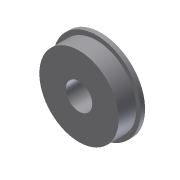
# Autodesk Inventor part: 375 ID 1125 OD flanged
Saved by Autodesk Inventor 2013 (Build 170138000, 138)
## iProperties
Created: 2011-07-15
Part Number: 375 ID 1125 OD flanged
Document SubType Name: Modeling
Designer: Dan Niemitalo
Density: 4.77592 g/cm^3
Mass: 31.751 g
Surface Area: 28.0121 cm^2
Volume: 6.64815 cm^3
Material: Generic
Author: Dan Niemitalo
Autodesk Inventor part; units mm, degrees
ref_plane "YZ Plane" through (0, 0, 0) normal (1, 0, 0) x (0, 1, 0)
ref_plane "XZ Plane" through (0, 0, 0) normal (0, 1, 0) x (-1, 0, 0)
ref_plane "XY Plane" through (0, 0, 0) normal (0, 0, 1) x (1, 0, 0)
sketch "Sketch1" plane through (0, 0, 0) normal (0, 0, 1) x (1, 0, 0)
  circle A0 centre (0, 0) radius 4.7625
  circle A1 centre (0, 0) radius 14.2875
  dimension "d0" = 9.525
  dimension "d1" = 28.575
  constraints: 2 centre point, 2 coincident
  measures "d0" diameter of A0
  measures "d1" diameter of A1
extrude "Extrusion1" add sketch "Sketch1" along normal blind 6.35
sketch "Sketch2" plane through (0, 0, 0) normal (0, 0, -1) x (-1, 0, 0)
  circle A0 centre (0, 0) radius 4.7625 projected
  circle A1 centre (0, 0) radius 14.2875 projected
  circle A2 centre (0, 0) radius 15.875
  dimension "d4" = 31.75
  constraints: 1 centre point, 1 coincident
  measures "d4" diameter of A2
extrude "Extrusion2" add sketch "Sketch2" along normal blind 1.5748 contours A1 | A2
body "Solid1"
